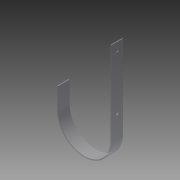
# Autodesk Inventor part: side guard
Saved by Autodesk Inventor 2014 SP1 (Build 180222100, 222)
## iProperties
Created: 2013-11-11
Part Number: side guard
Material: Polycarbonate, Clear
Document SubType Name: Modeling
Designer: RyanHughes
Density: 1.2 g/cm^3
Appearance: Polycarbonate - Clear
Author: RyanHughes
Autodesk Inventor part; units mm, degrees
note: some values were not read from the file. Chosen so that the rebuilt part matches the saved one: bend side of "Bend Part2".
ref_plane "YZ Plane" through (0, 0, 0) normal (1, 0, 0) x (0, 1, 0)
ref_plane "XZ Plane" through (0, 0, 0) normal (0, 1, 0) x (-1, 0, 0)
ref_plane "XY Plane" through (0, 0, 0) normal (0, 0, 1) x (1, 0, 0)
sketch "Sketch1" plane through (0, 0, 0) normal (0, 1, 0) x (-1, 0, 0)
  line L0 (152.4, -9.525) -> (-152.4, -9.525)
  line L1 (-152.4, -9.525) -> (-152.4, 9.525)
  line L2 (-152.4, 9.525) -> (152.4, 9.525)
  line L3 (152.4, 9.525) -> (152.4, -9.525)
  line L4 (152.4, -9.525) -> (-152.4, 9.525) construction
  line L5 (-152.4, -9.525) -> (152.4, 9.525) construction
  point P0 (0, 0)
  dimension "d0" = 19.05
  dimension "d1" = 304.8
  constraints: 12 end point, 2 midpoint, 2 parallel, 1 horizontal, 1 perpendicular
  measures "d0" distance of L0.end L1.end
  measures "d1" distance of L1.end L2.end
extrude "Extrusion1" add sketch "Sketch1" along normal blind 1.5875
sketch "Sketch2" plane through (0, 1.5875, 0) normal (0, 1, 0) x (1, 0, 0)
  line L0 (152.4, -9.525) -> (152.4, 9.525) projected
  line L1 (50.8, 36.3839) -> (50.8, -48.8029) construction
  line L2 (-50.8, 37.7294) -> (-50.8, -44.9073)
  line L3 (152.4, 9.525) -> (-152.4, 9.525) projected
  line L4 (-152.4, 9.525) -> (-152.4, -9.525) projected
  line L5 (-152.4, -9.525) -> (152.4, -9.525) projected
  line L6 (152.4, -9.525) -> (152.4, 9.525) projected
  line L7 (-152.4, 9.525) -> (50.8, -9.525) construction
  line L8 (50.8, 9.525) -> (-152.4, -9.525) construction
  point P0 (0, 0)
  point P1 (-50.8, 0)
  dimension "d4" = 101.6
  constraints: 8 end point, 5 point on line, 2 parallel, 1 midpoint
  measures "d4" distance between parallel lines of L0 L1
bend part "Bend Part2" radius 42.8509 angle 180 line through (-50.8, 1.5875, -37.7294) along (0, 0, 1) centre toward (0, 1, 0) moving side (1, 0, 0) both sides yes
sketch "Sketch3" plane through (-6.3616, 44.4384, -9.525) normal (1, 0, 0) x (0, 0, -1)
  line L0 (-19.05, 0) -> (0, 0) projected
  line L1 (0, 135.89) -> (-19.05, 135.89) projected
  line L2 (-19.05, 135.89) -> (-19.05, 0) projected
  circle A0 centre (-9.525, 123.19) radius 2.2225
  line L3 (-19.05, 0) -> (0, 135.89) construction
  line L4 (-19.05, 135.89) -> (0, 0) construction
  line L5 (-9.525, 0) -> (-9.525, 135.89) construction
  circle A1 centre (-9.525, 34.29) radius 2.2225
  point P0 (-9.525, -44.4384)
  dimension "d9" = 4.445
  dimension "d10" = 12.7
  dimension "d13" = 88.9
  constraints: 6 end point, 2 centre point, 2 midpoint, 1 point on line, 1 vertical, 2 other
  measures "d9" diameter of A0
  measures "d10" distance from line of L1 A0.centre
  measures "d13" distance of A0.centre A1.centre
extrude "Extrusion2" cut sketch "Sketch3" against normal blind 1.5875
body "Solid1"
